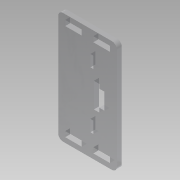
# Autodesk Inventor part: Front_wall
Saved by Autodesk Inventor 2016 (Build 200138000, 138)
## iProperties
Created: 2015-06-25
Part Number: Front_wall
Material: Generic
Document SubType Name: Modeling
Designer: Openlab
Density: 1 g/cm^3
Appearance: Polycarbonate - Clear
Author: Openlab
Autodesk Inventor part; units mm, degrees
ref_plane "YZ Plane" through (0, 0, 0) normal (1, 0, 0) x (0, 1, 0)
ref_plane "XZ Plane" through (0, 0, 0) normal (0, 1, 0) x (-1, 0, 0)
ref_plane "XY Plane" through (0, 0, 0) normal (0, 0, 1) x (1, 0, 0)
sketch "Sketch1" plane through (0, 0, 0) normal (0, 1, 0) x (-1, 0, 0)
  line L0 (17.75, -20.2435) -> (17.75, -42.6397) construction
  line L1 (13.2323, -33.7) -> (6.4845, -33.7) construction
  line L2 (35.5, -64.4) -> (35.5, -3)
  line L3 (0, -3) -> (0, -64.4)
  line L4 (32.5, 0) -> (3, 0)
  line L5 (3, -67.4) -> (32.5, -67.4)
  line L6 (16, -20.2) -> (14.2, -20.2)
  line L7 (14.2, -20.2) -> (14.2, -13.2)
  line L8 (14.2, -13.2) -> (16, -13.2)
  line L9 (16, -13.2) -> (16, -20.2)
  line L10 (31.25, -3) -> (21.25, -3)
  line L11 (21.25, -3) -> (21.25, -6.2)
  line L12 (21.25, -6.2) -> (31.25, -6.2)
  line L13 (31.25, -6.2) -> (31.25, -3)
  line L14 (14.25, -3) -> (4.25, -3)
  line L15 (4.25, -3) -> (4.25, -6.2)
  line L16 (4.25, -6.2) -> (14.25, -6.2)
  line L17 (14.25, -6.2) -> (14.25, -3)
  line L18 (31.25, -61.2) -> (21.25, -61.2)
  line L19 (21.25, -61.2) -> (21.25, -64.4)
  line L20 (21.25, -64.4) -> (31.25, -64.4)
  line L21 (31.25, -64.4) -> (31.25, -61.2)
  line L22 (14.25, -61.2) -> (4.25, -61.2)
  line L23 (4.25, -61.2) -> (4.25, -64.4)
  line L24 (4.25, -64.4) -> (14.25, -64.4)
  line L25 (14.25, -64.4) -> (14.25, -61.2)
  line L26 (10.7, -28.7) -> (7.5, -28.7)
  line L27 (7.5, -28.7) -> (7.5, -38.7)
  line L28 (7.5, -38.7) -> (10.7, -38.7)
  line L29 (10.7, -28.7) -> (10.7, -26.2)
  line L30 (10.7, -26.2) -> (13.9, -26.2)
  line L31 (13.9, -26.2) -> (13.9, -41.2)
  line L32 (13.9, -41.2) -> (10.7, -41.2)
  line L33 (10.7, -41.2) -> (10.7, -38.7)
  arc A0 (35.5, -3) -> (32.5, 0) centre (32.5, -3) ccw
  arc A1 (32.5, -67.4) -> (35.5, -64.4) centre (32.5, -64.4) ccw
  arc A2 (0, -64.4) -> (3, -67.4) centre (3, -64.4) ccw
  arc A3 (3, 0) -> (0, -3) centre (3, -3) ccw
  line L34 (16, -47.2) -> (14.2, -47.2)
  line L35 (14.2, -47.2) -> (14.2, -54.2)
  line L36 (14.2, -54.2) -> (16, -54.2)
  line L37 (16, -54.2) -> (16, -47.2)
  point P0 (0, 0)
  dimension "d22" = 7
  dimension "d24" = 1.8
  dimension "d27" = 10
  dimension "d28" = 3.2
  dimension "d30" = 3
  dimension "d31" = 7
  dimension "d33" = 10
  dimension "d34" = 15
  dimension "d35" = 6
  dimension "d39" = 7
  dimension "d52" = 35.5
  dimension "d53" = 4.25
  dimension "d54" = 7.5
  dimension "d55" = 3.5
  dimension "d56" = 55
  constraints: 76 end point, 15 parallel, 12 perpendicular, 10 point on line, 9 horizontal, 8 point on circle, 8 tangent, 7 equal length, 4 centre point, 3 equal radius, 2 vertical, 1 collinear, 6 other
  measures "d22" distance of L8.end L6.start
  measures "d24" distance of L7.end L8.end
  measures "d27" distance of L11.end L12.end
  measures "d28" distance of L14.end L15.end
  measures "d30" distance between parallel lines of L5 L24
  measures "d31" distance between parallel lines of L17 L11
  measures "d33" distance of L26.end L27.end
  measures "d34" distance of L30.end L31.end
  measures "d35" diameter of A0
  measures "d39" distance between parallel lines of L8 L12
  measures "d52" distance between parallel lines of L3 L2
  measures "d53" distance between parallel lines of L3 L15
  measures "d54" distance between parallel lines of L3 L27
  measures "d55" distance between parallel lines of L29 L7
  measures "d56" distance between parallel lines of L18 L12
extrude "Extrusion1" add sketch "Sketch1" along normal blind 3
body "Solid1"
